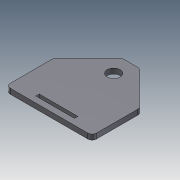
# Autodesk Inventor part: voetplaat poot
Saved by Autodesk Inventor 2015 (Build 190159000, 159)
## iProperties
Created: 2007-07-03
Part Number: voetplaat poot
Material: Steel, Mild
Document SubType Name: Sheet Metal
Designer: kurt
Manufacturer: Standard
Standards Organization: Custom
Density: 1 g/cm^3
Sheet Metal Rule: Default
Appearance: Steel
Author: kurt
Autodesk Inventor part; units mm, degrees
ref_plane "YZ Plane" through (0, 0, 0) normal (1, 0, 0) x (0, 1, 0)
ref_plane "XZ Plane" through (0, 0, 0) normal (0, 1, 0) x (-1, 0, 0)
sketch "Sketch1" plane through (0, 0, 0) normal (0, 0, 1) x (1, 0, 0)
  line L0 (-50, 0) -> (50, 0)
  line L1 (50, 0) -> (50, 55)
  line L2 (10, 95) -> (-10, 95)
  line L3 (-50, 55) -> (-50, 0)
  line L4 (-50, 55) -> (-10, 95)
  line L5 (50, 55) -> (10, 95)
  point P0 (0, 0)
  point P1 (50, 95)
  point P2 (-50, 95)
  point P3 (0, 0)
  dimension "d2" = 95
  dimension "d3" = 100
  dimension "d4" = 40
  dimension "d5" = 40
  dimension "d6" = 40
  dimension "d7" = 40
  measures "d2" distance of L0.end point (50, 95)
  measures "d3" distance of L0.start L0.end
  measures "d4" distance of L3.start point (-50, 95)
  measures "d5" distance of L2.end point (-50, 95)
  measures "d6" distance of L1.end point (50, 95)
  measures "d7" distance of L2.start point (50, 95)
extrude "Plate1" add sketch "Sketch1" along normal blind 6
hole "Hole1" at (0, 75, 6) direction (0, 0, -1) diameter 15 depth 6 tip angle 118
fillet "Corner Round1" radius 5 6 edges at (-50, 0, 3) (50, 0, 3) (50, 55, 3) (10, 95, 3) (-10, 95, 3) (-50, 55, 3)
ref_plane "Work Plane1" through (0, 0, 6) normal (1, 0, 0) x (0, 0, -1)
sketch "Sketch2" plane through (-45, 0, 6) normal (0, 0, 1) x (1, 0, 0)
  circle A0 centre (45, 75) radius 7.5 projected
  line L0 (22.5, 11) -> (67.5, 11)
  line L1 (67.5, 11) -> (67.5, 7)
  line L2 (67.5, 7) -> (22.5, 7)
  line L3 (22.5, 7) -> (22.5, 11)
  point P0 (0, 0)
  dimension "d19" = 4
  dimension "d20" = 45
  dimension "d21" = 7
  dimension "d22" = 22.5
  constraints: 8 end point, 2 parallel, 1 horizontal, 1 perpendicular
  measures "d19" distance of L0.end L1.end
  measures "d20" distance of L0.start L0.end
  measures "d21" vertical distance of point (0, 0) L2.end
  measures "d22" horizontal distance of A0.centre L0.end
extrude "Cut1" cut sketch "Sketch2" against normal blind 6 contours L0 L1 L2 L3
equation "\"d16\" = Thickness"
equation "\"d23\" = Thickness"
equation "\"d5\" = d4"
equation "\"d6\" = d4"
equation "\"d7\" = d6"
equation "\"BendReliefWidth\" = Thickness"
equation "\"CornerReliefSize\" = 4 * Thickness"
equation "\"MinimumRemnant\" = 2 * Thickness"
equation "\"TransitionRadius\" = BendRadius"
equation "\"d8\" = BendRadius"
equation "\"JacobiRadiusSize\" = Thickness"
equation "\"GapSize\" = Thickness"
equation "\"Thickness\" = 6"
equation "\"BendRadius\" = 0.001"
body "Solid1"
